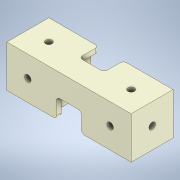
# Autodesk Inventor part: CornerPiece
Saved by Autodesk Inventor 2022.1 (Build 261234020, 234B)
## iProperties
Created: 2021-07-20
Part Number: CornerPiece
Material: ABS Plastic
Document SubType Name: Modeling
Designer: scb72
Density: 1.06 g/cm^3
Appearance: Smooth - White
Author: scb72
Autodesk Inventor part; units mm, degrees
ref_plane "YZ Plane" through (0, 0, 0) normal (1, 0, 0) x (0, 1, 0)
ref_plane "XZ Plane" through (0, 0, 0) normal (0, 1, 0) x (-1, 0, 0)
ref_plane "XY Plane" through (0, 0, 0) normal (0, 0, 1) x (1, 0, 0)
sketch "Sketch1" plane through (0, 0, 0) normal (0, 0, 1) x (1, 0, 0)
  line L0 (-13.5, -13.5) -> (13.5, -13.5)
  line L1 (13.5, -13.5) -> (13.5, 13.5)
  line L2 (13.5, 13.5) -> (-13.5, 13.5)
  line L3 (-13.5, 13.5) -> (-13.5, -13.5)
  line L4 (-13.5, -13.5) -> (13.5, 13.5) construction
  line L5 (13.5, -13.5) -> (-13.5, 13.5) construction
  point P0 (0, 0)
  dimension "d0" = 27
  dimension "d1" = 27
  constraints: 12 end point, 2 midpoint, 2 parallel, 1 horizontal, 1 perpendicular
  measures "d0" distance of L1.end L2.end
  measures "d1" distance of L2.end L0.start
extrude "Extrusion1" add sketch "Sketch1" along normal blind 27
sketch "Sketch2" plane through (13.5, -13.5, 0) normal (1, 0, 0) x (0, 0, -1)
  line L0 (0, 0) -> (-27, 0) projected
  line L1 (0, 0) -> (0, 27) projected
  point P0 (0, 13.5)
  point P1 (-13.5, 13.5)
  dimension "d4" = 13.5
  dimension "d5" = 13.5
  measures "d4" distance from line of L0 point (-13.5, 13.5)
  measures "d5" distance from line of L1 point (-13.5, 13.5)
sketch "Sketch3" plane through (-13.5, 13.5, 0) normal (0, 1, 0) x (1, 0, 0)
  line L0 (0, 0) -> (0, -27) projected
  line L1 (27, -27) -> (0, -27) projected
  point P0 (13.5, 0)
  point P1 (13.5, -13.5)
  dimension "d6" = 13.5
  dimension "d7" = 13.5
  measures "d6" distance from line of L0 point (13.5, -13.5)
  measures "d7" distance from line of L1 point (13.5, -13.5)
sketch "Sketch4" plane through (0, 0, 27) normal (0, 0, 1) x (1, 0, 0)
  line L0 (13.5, 13.5) -> (-13.5, 13.5) projected
  line L1 (-13.5, 13.5) -> (-13.5, -13.5) projected
  point P0 (0, 0)
  point P1 (0, 0)
  dimension "d8" = 13.5
  dimension "d9" = 13.5
  measures "d8" distance from line of L0 point (0, 0)
  measures "d9" distance from line of L1 point (0, 0)
hole "Hole1" at (0, 0, 27) direction (0, 0, -1) diameter 3.2 depth 15 tip angle 118 counterbore diameter 4.2 counterbore depth 5.5
hole "Hole2" at (0, 13.5, 13.5) direction (0, -1, 0) diameter 3.2 depth 15 tip angle 118 counterbore diameter 4.2 counterbore depth 5.5
hole "Hole3" at (13.5, 0, 13.5) direction (-1, 0, 0) diameter 3.2 depth 15 tip angle 118 counterbore diameter 4.2 counterbore depth 5.5
sketch "Sketch5" plane through (-13.5, -13.5, 0) normal (-1, 0, 0) x (0, 0, 1)
  circle A0 centre (6, 6) radius 1.6 projected
  line L0 (2.7957, 6) -> (4.3979, 8.775)
  line L1 (4.3979, 8.775) -> (7.6021, 8.775)
  line L2 (7.6021, 8.775) -> (9.2043, 6)
  line L3 (9.2043, 6) -> (7.6021, 3.225)
  line L4 (7.6021, 3.225) -> (4.3979, 3.225)
  line L5 (4.3979, 3.225) -> (2.7957, 6)
  point P0 (0, 13.5)
  dimension "d31" = 5.55
  constraints: 12 end point, 1 coincident, 13 other
  measures "d31" distance between parallel lines of L1 L4
extrude "Extrusion2" [suppressed]
sketch "Sketch6" plane through (0, 0, 0) normal (0, 0, -1) x (-1, 0, 0)
  circle A0 centre (0, 0) radius 1.6 projected
  line L0 (0, 3.2043) -> (2.775, 1.6021)
  line L1 (2.775, 1.6021) -> (2.775, -1.6021)
  line L2 (2.775, -1.6021) -> (0, -3.2043)
  line L3 (0, -3.2043) -> (-2.775, -1.6021)
  line L4 (-2.775, -1.6021) -> (-2.775, 1.6021)
  line L5 (-2.775, 1.6021) -> (0, 3.2043)
  point P0 (0, 0)
  dimension "d34" = 5.55
  constraints: 12 end point, 1 coincident, 13 other
  measures "d34" distance between parallel lines of L4 L1
extrude "Extrusion3" [suppressed]
sketch "Sketch7" plane through (-13.5, -13.5, 0) normal (0, -1, 0) x (1, 0, 0)
  circle A0 centre (10, 10) radius 1.6 projected
  line L0 (6.7957, 10) -> (8.3979, 12.775)
  line L1 (8.3979, 12.775) -> (11.6021, 12.775)
  line L2 (11.6021, 12.775) -> (13.2043, 10)
  line L3 (13.2043, 10) -> (11.6021, 7.225)
  line L4 (11.6021, 7.225) -> (8.3979, 7.225)
  line L5 (8.3979, 7.225) -> (6.7957, 10)
  point P0 (13.5, 0)
  dimension "d37" = 5.55
  constraints: 12 end point, 1 coincident, 13 other
  measures "d37" distance between parallel lines of L1 L4
extrude "Extrusion4" [suppressed]
sketch "Sketch23" plane through (-13.5, -13.5, 0) normal (-1, 0, 0) x (0, 0, 1)
  line L0 (0, 27) -> (0, 0) projected
  line L1 (0, 0) -> (27, 0) projected
  line L2 (27, 27) -> (27, 0) projected
  line L3 (0, 27) -> (27, 27) projected
  line L4 (24, 3) -> (3, 3)
  line L5 (3, 3) -> (3, 24)
  line L6 (3, 24) -> (24, 24)
  line L7 (24, 24) -> (24, 3)
  line L8 (24, 3) -> (24, 0)
  line L9 (3, 24) -> (0, 24)
  point P0 (0, 13.5)
  dimension "d77" = 3
  constraints: 12 end point, 2 perpendicular, 2 point on line, 3 other
  measures "d77" distance between parallel lines of L2 L7
extrude "Extrusion16" add sketch "Sketch23" along normal blind 13 contours L3 L2 L1 L8 L7 L6 L9 L0
mirror "Mirror1" about plane through (-26.5, 0, 13.5) normal (-1, 0, 0)
sketch "Sketch24" plane through (13.5, 13.5, 27) normal (0, 1, 0) x (1, 0, 0)
  line L0 (0, 27) -> (-80, 27) projected
  line L1 (-32, 39.5) -> (-48, 39.5)
  line L2 (-48, 39.5) -> (-48, 14.5)
  line L3 (-48, 14.5) -> (-32, 14.5)
  line L4 (-32, 14.5) -> (-32, 39.5)
  line L5 (-32, 39.5) -> (-48, 14.5) construction
  line L6 (-48, 39.5) -> (-32, 14.5) construction
  point P0 (-13.5, 27)
  point P1 (-40, 27)
  dimension "d82" = 16
  dimension "d83" = 12.5
  constraints: 12 end point, 3 midpoint, 2 parallel, 1 horizontal, 1 perpendicular
  measures "d82" distance of L1.start L1.end
  measures "d83" distance between parallel lines of L0 L3
extrude "Extrusion17" cut sketch "Sketch24" against normal blind 20
sketch "Sketch25" plane through (-13.5, -13.5, 24) normal (0, 0, -1) x (-1, 0, 0)
  line L0 (5, -12.5) -> (21, -12.5)
  line L1 (21, -12.5) -> (21, 12.5)
  line L2 (21, 12.5) -> (5, 12.5)
  line L3 (5, 12.5) -> (5, -12.5)
  line L4 (0, 0) -> (26, 0) projected
  line L5 (5, -12.5) -> (21, 12.5) construction
  line L6 (21, -12.5) -> (5, 12.5) construction
  point P0 (-13.5, 13.5)
  point P1 (13, 0)
  dimension "d86" = 16
  dimension "d87" = 12.5
  constraints: 12 end point, 3 midpoint, 2 parallel, 1 horizontal, 1 perpendicular
  measures "d86" distance of L1.end L2.end
  measures "d87" distance between parallel lines of L4 L2
extrude "Extrusion18" cut sketch "Sketch25" against normal blind 20
fillet "Fillet1" radius 2 8 edges at (-34.5, -13.5, 25.5) (-18.5, 12, 0) (-34.5, 12, 0) (-34.5, 12, 12.5) (-18.5, 12, 12.5) (-18.5, -1, 25.5) (-18.5, -13.5, 25.5) (-34.5, -1, 25.5)
body "Solid1"
